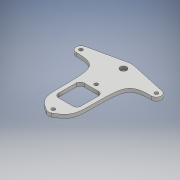
# Autodesk Inventor part: Corpo_Suporte_4_Cabos_Modelo4
Saved by Autodesk Inventor 2018 (Build 220112000, 112)
## iProperties
Created: 2021-08-09
Part Number: Corpo_Suporte_4_Cabos_Modelo4
Material: Generic
Document SubType Name: Modeling
Designer: L08619
Density: 1 g/cm^3
Appearance: Default
Author: L08619
Autodesk Inventor part; units mm, degrees
ref_plane "YZ Plane" through (0, 0, 0) normal (1, 0, 0) x (0, 1, 0)
ref_plane "XZ Plane" through (0, 0, 0) normal (0, 1, 0) x (-1, 0, 0)
ref_plane "XY Plane" through (0, 0, 0) normal (0, 0, 1) x (1, 0, 0)
sketch "Sketch2" plane through (0, 0, 0) normal (0, 0, 1) x (1, 0, 0)
  circle A0 centre (-235, 0) radius 11
  circle A1 centre (235, 0) radius 11
  circle A2 centre (0, -407.032) radius 11
  line L0 (0, -130) -> (0, -100) construction
  line L1 (0, 0) -> (0, 30) construction
  circle A3 centre (0, 30) radius 20
  line L2 (0, 201.7397) -> (0, -386.4818)
  line L3 (-241.4425, 29.3001) -> (-21.4752, 77.6669)
  arc A4 (21.4752, 77.6669) -> (-21.4752, 77.6669) centre (0, -20) ccw
  line L4 (21.4752, 77.6669) -> (241.4425, 29.3001)
  circle A5 centre (0, -140) radius 11
  line L5 (-45, -170) -> (45, -170)
  line L6 (70, -195) -> (70, -305)
  line L7 (45, -330) -> (-45, -330)
  line L8 (-70, -305) -> (-70, -195)
  arc A6 (-14.2105, -433.4528) -> (14.2105, -433.4528) centre (0, -407.032) ccw
  arc A7 (235, -30) -> (241.4425, 29.3001) centre (235, 0) ccw
  arc A8 (-241.4425, 29.3001) -> (-235, -30) centre (-235, 0) ccw
  line L9 (-235, -30) -> (-210, -30) construction
  line L10 (-210, -30) -> (-105, -30) construction
  line L11 (-105, -30) -> (-95, -110) construction
  line L12 (-95, -110) -> (-95, -325) construction
  line L13 (-95, -325) -> (-95, -390) construction
  line L14 (-95, -390) -> (-14.2105, -433.4528) construction
  spline S0 degree 4 poles (-235, -30) (-210, -30) (-105, -30) (-95, -110) (-95, -325) (-95, -390) (-14.2105, -433.4528) knots 1 1 1 1 1 2 3 4 4 4 4 4
  arc A9 (-45, -170) -> (-70, -195) centre (-45, -195) ccw
  arc A10 (70, -195) -> (45, -170) centre (45, -195) ccw
  arc A11 (45, -330) -> (70, -305) centre (45, -305) ccw
  arc A12 (-70, -305) -> (-45, -330) centre (-45, -305) ccw
  line L15 (235, -30) -> (210, -30) construction
  line L16 (210, -30) -> (105, -30) construction
  line L17 (105, -30) -> (95, -110) construction
  line L18 (95, -110) -> (95, -325) construction
  line L19 (95, -325) -> (95, -390) construction
  line L20 (95, -390) -> (14.2105, -433.4528) construction
  spline S1 degree 4 poles (235, -30) (210, -30) (105, -30) (95, -110) (95, -325) (95, -390) (14.2105, -433.4528) knots 1 1 1 1 1 2 3 4 4 4 4 4
  point P0 (-17.2975, -383.8099)
  point P1 (-17.2975, -383.8099)
  point P2 (70, -330)
  point P3 (70, -170)
  point P4 (-70, -330)
  dimension "d24" = 22
  dimension "d25" = 22
  dimension "d31" = 22
  dimension "d32" = 407.032
  dimension "d33" = 0
  dimension "d44" = 30
  dimension "d46" = 40
  dimension "d59" = 22
  dimension "d60" = 140
  dimension "d61" = 140
  dimension "d62" = 160
  dimension "d63" = 30
  dimension "d64" = 60
  dimension "d65" = 60
  dimension "d66" = 60
  dimension "d67" = 25
  dimension "d68" = 100
  dimension "d69" = 20
  dimension "d72" = 470
  dimension "d75" = 25
  dimension "d76" = 30
  dimension "d77" = 190
  dimension "d78" = 210
  dimension "d79" = 30
  dimension "d80" = 80
  dimension "d81" = 215
  dimension "d82" = 65
  constraints: 19 end point, 16 point on circle, 13 centre point, 12 tangent, 10 point on line, 7 symmetric about line, 5 coincident, 4 vertical, 3 equal radius, 2 parallel, 1 horizontal, 1 horizontal alignment, 1 perpendicular, 11 other
  measures "d24" diameter of A0
  measures "d25" diameter of A1
  measures "d31" diameter of A2
  measures "d32" vertical distance of A1.centre A2.centre
  measures "d33" vertical distance of L1.start A1.centre
  measures "d44" distance of L1.start L1.end
  measures "d46" diameter of A3
  measures "d59" diameter of A5
  measures "d60" vertical distance of A1.centre A5.centre
  measures "d61" distance of point (70, -330) point (-70, -330)
  measures "d62" distance of point (70, -170) point (70, -330)
  measures "d63" distance from line of A5.centre L5
  measures "d64" diameter of A6
  measures "d65" diameter of A7
  measures "d66" diameter of A8
  measures "d67" radius of A9
  measures "d68" radius of A4
  measures "d69" distance of L1.start A4.centre
  measures "d72" diameter of A0.centre L2
  measures "d75" horizontal distance of A0.centre L9.end
  measures "d76" vertical distance of A0.centre L9.end
  measures "d77" diameter of L11.end L2
  measures "d78" diameter of L10.end L2
  measures "d79" vertical distance of A0.centre L10.end
  measures "d80" vertical distance of L10.end L11.end
  measures "d81" distance of L11.end L12.end
  measures "d82" distance of L13.end L12.end
extrude "Extrusion1" add sketch "Sketch2" along normal mid plane 22.22
body "Solid1"
